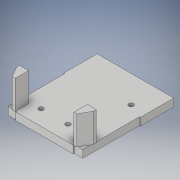
# Autodesk Inventor part: Base
Saved by Autodesk Inventor 2018 (Build 220112000, 112)
## iProperties
Created: 2018-11-07
Part Number: Base
Material: Generic
Document SubType Name: Modeling
Designer: kjy5515
Density: 1 g/cm^3
Appearance: Default
Author: kjy5515
Autodesk Inventor part; units mm, degrees
ref_plane "YZ Plane" through (0, 0, 0) normal (1, 0, 0) x (0, 1, 0)
ref_plane "XZ Plane" through (0, 0, 0) normal (0, 1, 0) x (-1, 0, 0)
ref_plane "XY Plane" through (0, 0, 0) normal (0, 0, 1) x (1, 0, 0)
sketch "Sketch1" plane through (0, 0, 0) normal (0, 1, 0) x (-1, 0, 0)
  line L0 (40, 47.5) -> (-40, 47.5)
  line L1 (-40, 47.5) -> (-40, -47.5)
  line L2 (-40, -47.5) -> (40, -47.5)
  line L3 (40, -47.5) -> (40, 47.5)
  line L4 (40, 47.5) -> (-40, -47.5) construction
  line L5 (-40, 47.5) -> (40, -47.5) construction
  point P0 (0, 0)
  dimension "d0" = 80
  dimension "d1" = 95
  constraints: 12 end point, 2 midpoint, 2 parallel, 1 horizontal, 1 perpendicular
  measures "d0" distance of L2.end L1.end
  measures "d1" distance of L1.end L0.end
extrude "Extrusion1" add sketch "Sketch1" along normal blind 8
sketch "Sketch2" plane through (0, 8, 0) normal (0, 1, 0) x (1, 0, 0)
  line L0 (0, 0) -> (0, 19)
  line L1 (0, 19) -> (24, 19)
  line L2 (0, 0) -> (0, -31.5)
  line L3 (0, -31.5) -> (-19.5, -31.5)
  line L4 (0, -31.5) -> (8.5, -31.5)
  circle A0 centre (8.5, -31.5) radius 2.5
  circle A1 centre (-19.5, -31.5) radius 2.5
  circle A2 centre (24, 19) radius 2.5
  dimension "d4" = 19
  dimension "d5" = 24
  dimension "d6" = 31.5
  dimension "d7" = 19.5
  dimension "d8" = 8.5
  dimension "d9" = 5
  dimension "d10" = 5
  dimension "d11" = 5
  constraints: 10 end point, 3 centre point, 3 coincident, 2 perpendicular, 2 vertical, 1 horizontal
  measures "d4" distance of L0.start L0.end
  measures "d5" distance of L0.end L1.end
  measures "d6" distance of L0.start L2.end
  measures "d7" distance of L2.end L3.end
  measures "d8" distance of L2.end L4.end
  measures "d9" diameter of A0
  measures "d10" diameter of A1
  measures "d11" diameter of A2
extrude "Extrusion2" cut sketch "Sketch2" against normal blind 8
sketch "Sketch4" plane through (0, 8, 0) normal (0, 1, 0) x (1, 0, 0)
  line L0 (-40, -47.5) -> (40, -47.5) projected
  line L1 (-40, -47.5) -> (-40, -36.5)
  line L2 (-40, -36.5) -> (-33.6491, -47.5)
  line L3 (-33.6491, -47.5) -> (-30.6491, -47.5)
  line L4 (-30.6491, -47.5) -> (-30.6491, -33.5)
  line L5 (-30.6491, -33.5) -> (-40, -33.5)
  line L6 (-40, 47.5) -> (-40, -47.5) projected
  line L7 (-40, -36.5) -> (-40, -33.5)
  line L8 (0, -20.8898) -> (0, -30.7247)
  line L9 (40, -47.5) -> (40, -36.5)
  line L10 (40, -36.5) -> (33.6491, -47.5)
  line L11 (33.6491, -47.5) -> (30.6491, -47.5)
  line L12 (30.6491, -47.5) -> (30.6491, -33.5)
  line L13 (30.6491, -33.5) -> (40, -33.5)
  line L14 (40, -36.5) -> (40, -33.5)
  point P0 (0, 0)
  point P1 (-32.5008, -49.4891)
  point P2 (32.5008, -49.4891)
  dimension "d14" = 11
  dimension "d15" = 30
  dimension "d16" = 3
  dimension "d17" = 14
  constraints: 26 end point, 6 symmetric about line, 3 perpendicular, 3 point on line, 3 vertical
  measures "d14" distance of L0.start L1.end
  measures "d15" angle of L1 L2
  measures "d16" distance of L2.end L3.end
  measures "d17" distance of L3.end L4.end
extrude "Extrusion3" add sketch "Sketch4" along normal blind 30 contours L2 L6 L5 L4 L0 | L12 L13 L14 L10 L0
sketch "Sketch5" plane through (0, 0, 0) normal (0, -1, 0) x (1, 0, 0)
  circle A0 centre (-19.5, 31.5) radius 2.5 projected
  circle A1 centre (8.5, 31.5) radius 2.5 projected
  circle A2 centre (24, -19) radius 2.5 projected
  line L0 (-40, 47.5) -> (40, 47.5) projected
  line L1 (-40, -47.5) -> (-40, 47.5) projected
  line L2 (40, -47.5) -> (-40, -47.5) projected
  line L3 (40, 47.5) -> (40, -47.5) projected
  line L4 (40, 47.5) -> (40, -12.5)
  line L5 (40, -12.5) -> (39, -12.5)
  line L6 (39, -12.5) -> (39, 47.5)
  line L7 (33.6491, 47.5) -> (40, 47.5) projected
  line L8 (40, 47.5) -> (39, 47.5)
  line L9 (40, 47.5) -> (40, 46.5)
  line L10 (40, 47.5) -> (40, 36.5) projected
  line L11 (40, 46.5) -> (30, 46.5)
  line L12 (30, 46.5) -> (30, 47.5)
  line L13 (40, 47.5) -> (30, 47.5)
  line L14 (-30.6491, 47.5) -> (30.6491, 47.5) projected
  line L15 (0, 47.5) -> (0, 0)
  line L16 (-40, 47.5) -> (-40, -12.5)
  line L17 (-40, -12.5) -> (-39, -12.5)
  line L18 (-39, -12.5) -> (-39, 47.5)
  line L19 (-33.6491, 47.5) -> (-40, 47.5)
  line L20 (-40, 47.5) -> (-39, 47.5)
  line L21 (-40, 47.5) -> (-40, 46.5)
  line L22 (-40, 47.5) -> (-40, 36.5)
  line L23 (-40, 46.5) -> (-30, 46.5)
  line L24 (-30, 46.5) -> (-30, 47.5)
  line L25 (-40, 47.5) -> (-30, 47.5)
  dimension "d20" = 60
  dimension "d21" = 1
  dimension "d22" = 1
  dimension "d23" = 10
  constraints: 38 end point, 8 symmetric about line, 6 point on line, 4 perpendicular, 2 collinear, 1 midpoint, 1 vertical
  measures "d20" distance of L0.end L4.end
  measures "d21" distance of L4.end L5.end
  measures "d22" distance of L0.end L9.end
  measures "d23" distance of L9.end L11.end
extrude "Extrusion4" cut sketch "Sketch5" against normal blind 8 contours L0 L18 L23 L1 | L0 L24 L23 L18 | L23 L18 L17 L1 | L0 L6 L11 L12 | L5 L6 L11 L3 | L6 L0 L3 L11
body "Solid1"
